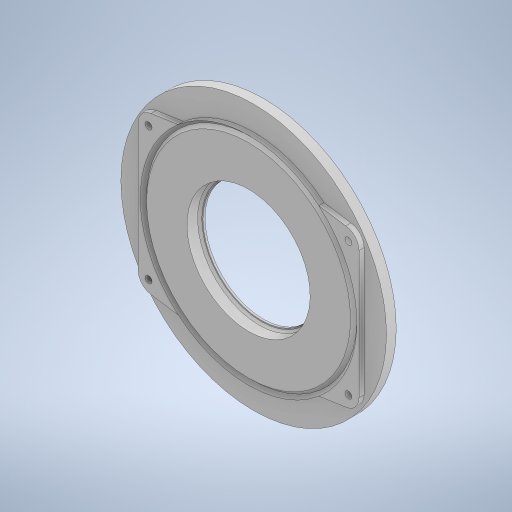
# Autodesk Inventor part: frame_rring2
Saved by Autodesk Inventor 2023.4 (Build 274418000, 418)
## iProperties
Created: 2023-11-26
Part Number: frame_rring2
Material: Generic
Document SubType Name: Modeling
Designer: aaron
Density: 1 g/cm^3
Appearance: Default
Author: aaron
Autodesk Inventor part; units mm, degrees
ref_plane "YZ Plane" through (0, 0, 0) normal (1, 0, 0) x (0, 1, 0)
ref_plane "XZ Plane" through (0, 0, 0) normal (0, 1, 0) x (-1, 0, 0)
ref_plane "XY Plane" through (0, 0, 0) normal (0, 0, 1) x (1, 0, 0)
sketch "Sketch1" plane through (0, 0, 0) normal (0, 0, 1) x (1, 0, 0)
  circle A0 centre (-47.0107, -31.3407) radius 4.8
  arc A1 (51.632, -32.6385) -> (49.9861, -35.1073) centre (47.0107, -31.3407) ccw
  arc A2 (51.632, -32.6385) -> (51.632, 32.6385) centre (0, 0) ccw
  arc A3 (49.9861, 35.1073) -> (51.632, 32.6385) centre (47.0107, 31.3407) ccw
  arc A4 (49.9861, 35.1073) -> (-42.369, 44) centre (0, 0) ccw
  line L0 (-42.369, 44) -> (-62, 44)
  line L1 (-62, 44) -> (-64, 42)
  line L2 (-64, 42) -> (-64, 0.1)
  arc A5 (0, -61.083) -> (49.9861, -35.1073) centre (0, 0) ccw
  circle A6 centre (0, 0) radius 48
  circle A7 centre (-58, 38) radius 3.825
  circle A8 centre (-47.0107, 31.3407) radius 4.8
  line L3 (0, 0) -> (-74.8823, 0)
  circle A9 centre (-58, -38) radius 3.825
  line L4 (-42.369, -44) -> (-62, -44)
  arc A10 (-42.369, -44) -> (49.9861, -35.1073) centre (0, 0) ccw
  line L5 (-62, -44) -> (-64, -42)
  line L6 (-64, -42) -> (-64, 0.1)
  constraints: 14 end point, 12 point on circle, 11 centre point, 4 symmetric about line, 1 horizontal, 2 other
extrude "Extrusion1" add sketch "Sketch1" along normal blind 4.8
sketch "Sketch5" plane through (0, 0, 4.8) normal (0, 0, 1) x (1, 0, 0)
  circle A0 centre (0, 0) radius 48 projected
  circle A1 centre (-47.0107, 31.3407) radius 4.8 projected
  circle A2 centre (0, 0) radius 61.5
  arc A3 (49.9861, 35.1073) -> (51.632, 32.6385) centre (47.0107, 31.3407) ccw projected
  circle A4 centre (47.0107, 31.3407) radius 1.6
  arc A5 (51.632, -32.6385) -> (49.9861, -35.1073) centre (47.0107, -31.3407) ccw projected
  circle A6 centre (47.0107, -31.3407) radius 1.6
  circle A7 centre (-47.0107, -31.3407) radius 4.8 projected
  circle A8 centre (-47.0107, -31.3407) radius 1.6
  circle A9 centre (-47.0107, 31.3407) radius 4.8 projected
  circle A10 centre (-47.0107, 31.3407) radius 1.6
  dimension "d14" = 123
  dimension "d41" = 3.2
  dimension "d42" = 3.2
  dimension "d43" = 3.2
  dimension "d44" = 3.2
  constraints: 5 centre point, 5 coincident
  measures "d14" diameter of A2
  measures "d41" diameter of A4
  measures "d42" diameter of A6
  measures "d43" diameter of A8
  measures "d44" diameter of A10
extrude "Extrusion5" add sketch "Sketch5" against normal up to surface (4.8 mm away) contours A1 | A2 | A7
sketch "Sketch8" plane through (0, 0, 0) normal (0, 0, -1) x (-1, 0, 0)
  circle A0 centre (0, 0) radius 48 projected
  circle A1 centre (0, 0) radius 29
  dimension "d30" = 58
  constraints: 1 centre point, 1 coincident
  measures "d30" diameter of A1
extrude "Extrusion8" add sketch "Sketch8" against normal up to surface (4.8 mm away)
sketch "Sketch9" plane through (0, 0, 0) normal (0, 0, -1) x (-1, 0, 0)
  circle A0 centre (0, 0) radius 29 projected
  circle A1 centre (0, 0) radius 27.5
  dimension "d33" = 1.5
  constraints: 1 centre point
  measures "d33" radial gap between concentric circles of A0 A1
extrude "Extrusion9" add sketch "Sketch9" against normal blind 1
chamfer "Chamfer3" distance 1 angle 45 1 edges at (29, 0, 1)
sketch "Sketch10" plane through (0, 0, 4.8) normal (0, 0, 1) x (1, 0, 0)
  circle A0 centre (0, 0) radius 29 projected
  circle A1 centre (-58, 38) radius 3.825 projected
  arc A2 (-42.968, -44) -> (-42.968, 44) centre (0, 0) ccw projected
  line L0 (-42.968, 44) -> (-62, 44) projected
  line L1 (-62, 44) -> (-64, 42) projected
  line L2 (-64, 42) -> (-64, -42) projected
  circle A3 centre (47.0107, 31.3407) radius 1.6 projected
  circle A4 centre (47.0107, -31.3407) radius 1.6 projected
  circle A5 centre (-47.0107, -31.3407) radius 1.6 projected
  circle A6 centre (-47.0107, 31.3407) radius 1.6 projected
  line L3 (-64, -42) -> (-62, -44) projected
  line L4 (-62, -44) -> (-42.968, -44) projected
  circle A7 centre (-58, -38) radius 3.825 projected
extrude "Extrusion10" add sketch "Sketch10" along normal blind 2.2
sketch "Sketch11" plane through (0, 0, 0) normal (0, 0, -1) x (-1, 0, 0)
  circle A0 centre (-47.0107, -31.3407) radius 1.6 projected
  circle A1 centre (-47.0107, -31.3407) radius 3
  circle A2 centre (-47.0107, 31.3407) radius 1.6 projected
  circle A3 centre (-47.0107, 31.3407) radius 3
  circle A4 centre (47.0107, 31.3407) radius 1.6 projected
  circle A5 centre (47.0107, 31.3407) radius 3
  circle A6 centre (47.0107, -31.3407) radius 1.6 projected
  circle A7 centre (47.0107, -31.3407) radius 3
  point P0 (0, 0)
  dimension "d45" = 6
  dimension "d46" = 6
  dimension "d47" = 6
  dimension "d48" = 6
  constraints: 4 centre point, 4 coincident
  measures "d45" diameter of A1
  measures "d46" diameter of A3
  measures "d47" diameter of A5
  measures "d48" diameter of A7
extrude "Extrusion11" cut sketch "Sketch11" against normal blind 4 contours A1 | A3 | A5 | A6 | A7
sketch "Sketch12" plane through (0, 0, 7) normal (0, 0, 1) x (1, 0, 0)
  circle A0 centre (0, 0) radius 48
  circle A1 centre (0, 0) radius 51
  dimension "d51" = 96
  dimension "d52" = 3
  constraints: 2 centre point, 1 coincident
  measures "d51" diameter of A0
  measures "d52" radial gap between concentric circles of A0 A1
extrude "Extrusion12" cut sketch "Sketch12" against normal blind 1.5
chamfer "Chamfer4" distance 1.5 angle 45 2 edges at (-51, 0, 5.5) (-48, 0, 5.5)
sketch "Sketch17" plane through (0, 0, 7) normal (0, 0, 1) x (1, 0, 0)
  circle A0 centre (0, 0) radius 61.5
  circle A1 centre (0, 0) radius 96.3014
  point P0 (-42.968, 44)
  constraints: 2 coincident, 1 centre point, 3 other
extrude "Extrusion15" cut sketch "Sketch17" against normal through all
sketch "Sketch19" plane through (0, 0, 0) normal (0, 0, -1) x (-1, 0, 0)
  circle A0 centre (-47.0107, -31.3407) radius 3 projected
  line L0 (0, 0) -> (-47.0107, -31.3407)
  line L1 (-47.0107, -31.3407) -> (-60.1837, -40.1228)
  circle A1 centre (0, 0) radius 65
  circle A2 centre (0, 0) radius 61.5 projected
  circle A3 centre (-54.0831, -36.0557) radius 2.05
  circle A4 centre (-54.0831, -36.0557) radius 4
  line L2 (-54.8676, -39.978) -> (-36.9294, -43.5656)
  line L3 (-58.0055, -35.2712) -> (-54.4179, -17.333)
  point P0 (-44.9634, -41.9588)
  point P1 (-56.0247, -25.367)
  point P2 (-58.0055, -35.2712)
  dimension "d67" = 130
  dimension "d69" = 8
  dimension "d68" = 4.1
  dimension "d70" = 45
  constraints: 8 end point, 2 coincident, 2 point on line, 2 symmetric about line, 1 centre point, 7 other
  measures "d68" diameter of A3
  measures "d70" angle of L1 L2
extrude "Extrusion16" add sketch "Sketch19" against normal up to surface (7 mm away) contours A2 A4 A1 A3 L1 | L1 A3 A1 A4 A2 | A2 L2 A1 A4 | A4 A1 L3 A2 | A4 L3 A1 | A1 A3 L1 A4 | L2 A4 A1 | A4 L1 A3 A1
sketch "Sketch20" plane through (0, 0, 7) normal (0, 0, 1) x (1, 0, 0)
  arc A0 (33.0898, 38.808) -> (-18.5896, 47.4913) centre (0, 0) ccw
  line L0 (45.7919, 36.955) -> (33.0898, 38.808)
  arc A1 (51.7244, 28.0563) -> (45.7919, 36.955) centre (44.9997, 30) ccw
  line L1 (48.5496, 15.6186) -> (51.7244, 28.0563)
  arc A2 (48.5496, -15.6186) -> (48.5496, 15.6186) centre (0, 0) ccw
  line L2 (51.7244, -28.0563) -> (48.5496, -15.6186)
  arc A3 (45.7919, -36.955) -> (51.7244, -28.0563) centre (44.9997, -30) ccw
  line L3 (33.0898, -38.808) -> (45.7919, -36.955)
  arc A4 (-18.5896, -47.4913) -> (33.0898, -38.808) centre (0, 0) ccw
  line L4 (-33.7876, -44) -> (-18.5896, -47.4913)
  line L5 (-62, -44) -> (-33.7876, -44)
  line L6 (-64, -42) -> (-62, -44)
  line L7 (-64, 42) -> (-64, -42)
  line L8 (-62, 44) -> (-64, 42)
  line L9 (-33.7876, 44) -> (-62, 44)
  line L10 (-18.5896, 47.4913) -> (-33.7876, 44)
  circle A5 centre (0, 0) radius 88.8325
  constraints: 22 end point, 10 point on circle, 6 centre point, 1 coincident
extrude "Extrusion17" cut sketch "Sketch20" against normal blind 2.4
sketch "Sketch21" plane through (0, 0, 0) normal (0, 0, -1) x (-1, 0, 0)
  circle A0 centre (0, 0) radius 78.6238
  circle A1 centre (0, 0) radius 61.5
  constraints: 2 centre point, 2 coincident
extrude "Extrusion18" cut sketch "Sketch21" against normal through all
sketch "Sketch22" plane through (0, 0, 0) normal (0, 0, -1) x (-1, 0, 0)
  circle A0 centre (0, 0) radius 61.5 projected
  circle A1 centre (0, 0) radius 27.5 projected
  circle A2 centre (0, 0) radius 62.5
  dimension "d77" = 1
  constraints: 1 centre point, 1 coincident
  measures "d77" radial gap between concentric circles of A2 A0
extrude "Extrusion19" add sketch "Sketch22" against normal up to surface (4.6 mm away) contours A2
sketch "Sketch23" plane through (0, 0, 7) normal (0, 0, 1) x (1, 0, 0)
  circle A0 centre (47.0107, 31.3407) radius 1.6 projected
  line L0 (48.5496, 15.6186) -> (51.7244, 28.0563) projected
  arc A1 (51.7244, 28.0563) -> (45.7919, 36.955) centre (44.9997, 30) ccw projected
  line L1 (45.7919, 36.955) -> (33.0898, 38.808) projected
  arc A2 (48.5496, 15.6186) -> (33.0898, 38.808) centre (0, 0) ccw projected
  line L2 (51.7244, -28.0563) -> (48.5496, -15.6186) projected
  arc A3 (33.0898, -38.808) -> (48.5496, -15.6186) centre (0, 0) ccw projected
  line L3 (33.0898, -38.808) -> (45.7919, -36.955) projected
  arc A4 (45.7919, -36.955) -> (51.7244, -28.0563) centre (44.9997, -30) ccw projected
  circle A5 centre (47.0107, -31.3407) radius 1.6 projected
  arc A6 (48.5496, -15.6186) -> (48.5496, 15.6186) centre (0, 0) ccw projected
  line L4 (51.9997, 39.8529) -> (51.9997, -52.1761)
  point P0 (51.9997, -30)
  point P1 (51.9997, 30)
  constraints: 2 end point, 1 tangent, 1 vertical
extrude "Extrusion20" add sketch "Sketch23" against normal up to surface (2.4 mm away) contours L0 A1 L4 A4 L2 A6
sketch "Sketch24" plane through (0, 0, 7) normal (0, 0, 1) x (1, 0, 0)
  line L0 (0, -84.8798) -> (-71.6508, -84.8798)
  line L1 (-71.6508, -84.8798) -> (-71.6508, 87.4797)
  line L2 (-71.6508, 87.4797) -> (0, 87.4797)
  line L3 (0, 87.4797) -> (0, -84.8798)
  point P0 (0, 0)
  constraints: 8 end point, 2 parallel, 1 horizontal, 1 perpendicular
extrude "Extrusion21" cut sketch "Sketch24" along normal through all both and the other way through all
mirror "Mirror1" about plane through (0, -84.8798, 7) normal (-1, 0, 0)
body "Solid1"
